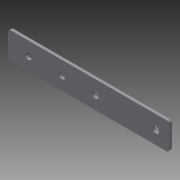
# Autodesk Inventor part: Connector_H2
Saved by Autodesk Inventor 2015 (Build 190159000, 159)
## iProperties
Created: 2015-04-22
Part Number: Connector_H2
Material: Generic
Document SubType Name: Modeling
Designer: krosie
Density: 1 g/cm^3
Appearance: Default
Author: krosie
Autodesk Inventor part; units mm, degrees
ref_plane "YZ Plane" through (0, 0, 0) normal (1, 0, 0) x (0, 1, 0)
ref_plane "XZ Plane" through (0, 0, 0) normal (0, 1, 0) x (-1, 0, 0)
ref_plane "XY Plane" through (0, 0, 0) normal (0, 0, 1) x (1, 0, 0)
sketch "Sketch4" plane through (0, 0, 0) normal (0, 1, 0) x (-1, 0, 0)
  line L0 (0, 0) -> (-120, 0)
  line L1 (-120, 0) -> (-120, -20)
  line L2 (-120, -20) -> (0, -20)
  line L3 (0, -20) -> (0, 0)
  circle A0 centre (-15, -10) radius 2.5
  circle A1 centre (-40, -10) radius 2.5
  circle A2 centre (-65, -10) radius 2.5
  circle A3 centre (-110, -10) radius 2.5
  dimension "d6" = 120
  dimension "d7" = 20
  dimension "d11" = 5
  dimension "d12" = 5
  dimension "d13" = 5
  dimension "d14" = 5
  dimension "d15" = 10
  dimension "d16" = 15
  dimension "d17" = 25
  dimension "d18" = 25
  constraints: 8 end point, 4 centre point, 3 perpendicular, 1 horizontal
  measures "d6" distance of L0.start L0.end
  measures "d7" distance of L0.end L1.end
  measures "d11" diameter of A0
  measures "d12" diameter of A1
  measures "d13" diameter of A2
  measures "d14" diameter of A3
  measures "d15" distance from line of L1 A3.centre
  measures "d16" distance from line of L3 A0.centre
  measures "d17" distance of A1.centre A0.centre
  measures "d18" distance of A2.centre A1.centre
extrude "Extrusion2" add sketch "Sketch4" along normal blind 2
fillet "Fillet2" radius 2 4 edges at (0, 1, -20) (0, 1, 0) (120, 1, 0) (120, 1, -20)
body "Solid3"
